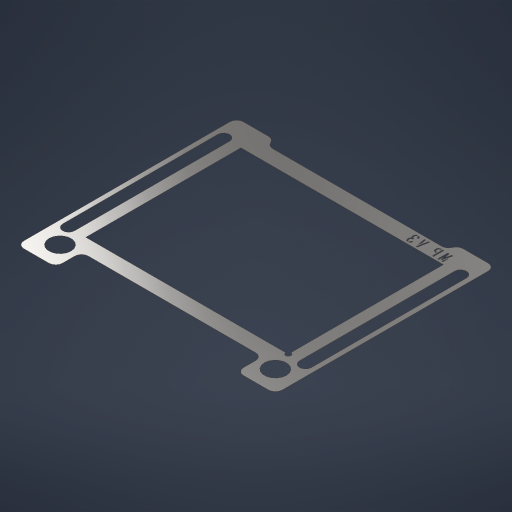
# Autodesk Inventor part: Module PCB Stencil - V3
Saved by Autodesk Inventor 2024 (Build 280153000, 153)
## iProperties
Created: 2022-06-23
Part Number: Module PCB Stencil - V3
Material: Stainless Steel
Document SubType Name: Modeling
Designer: Caleb
Density: 8 g/cm^3
Appearance: Semi-Polished
Author: Caleb
Autodesk Inventor part; units mm, degrees
ref_plane "YZ Plane" through (0, 0, 0) normal (1, 0, 0) x (0, 1, 0)
ref_plane "XZ Plane" through (0, 0, 0) normal (0, 1, 0) x (-1, 0, 0)
ref_plane "XY Plane" through (0, 0, 0) normal (0, 0, 1) x (1, 0, 0)
sketch "Sketch1" plane through (0, 0, 0) normal (0, 1, 0) x (-1, 0, 0)
  line L0 (-38.1, -34.925) -> (38.1, -34.925)
  line L1 (38.1, -34.925) -> (38.1, 34.925)
  line L2 (38.1, 34.925) -> (-38.1, 34.925)
  line L3 (-38.1, 34.925) -> (-38.1, -34.925)
  line L4 (-38.1, -34.925) -> (38.1, 34.925) construction
  line L5 (38.1, -34.925) -> (-38.1, 34.925) construction
  point P0 (0, 0)
  dimension "d0" = 76.2
  dimension "d1" = 69.85
  constraints: 12 end point, 2 midpoint, 2 parallel, 1 horizontal, 1 perpendicular
  measures "d0" distance of L2.end L1.end
  measures "d1" distance of L1.end L0.end
extrude "Extrusion1" add sketch "Sketch1" along normal blind 0.0508
sketch "Sketch2" plane through (0, 0.0508, 0) normal (0, 1, 0) x (1, 0, 0)
  line L0 (34.925, -22.86) -> (34.925, 22.86) construction
  line L1 (36.675, -22.86) -> (36.675, 22.86)
  line L2 (33.175, 22.86) -> (33.175, -22.86)
  arc A0 (33.175, -22.86) -> (36.675, -22.86) centre (34.925, -22.86) ccw
  arc A1 (36.675, 22.86) -> (33.175, 22.86) centre (34.925, 22.86) ccw
  line L3 (38.1, -34.925) -> (38.1, 34.925) projected
  line L4 (0, -11.2063) -> (0, 14.7333)
  line L5 (-34.925, -22.86) -> (-34.925, 22.86) construction
  line L6 (-36.675, -22.86) -> (-36.675, 22.86)
  line L7 (-33.175, 22.86) -> (-33.175, -22.86)
  arc A2 (-36.675, -22.86) -> (-33.175, -22.86) centre (-34.925, -22.86) ccw
  arc A3 (-33.175, 22.86) -> (-36.675, 22.86) centre (-34.925, 22.86) ccw
  line L8 (-38.1, -34.925) -> (38.1, -34.925) projected
  line L9 (-38.1, 34.925) -> (-38.1, -34.925) projected
  point P0 (0, 0)
  point P1 (34.925, 0)
  point P2 (-34.925, 0)
  point P3 (31.75, -28.575)
  point P4 (-31.75, -28.575)
  dimension "d4" = 3.5
  dimension "d5" = 3.175
  dimension "d6" = 45.72
  dimension "d14" = 6.35
  dimension "d15" = 6.35
  dimension "d16" = 6.35
  dimension "d17" = 6.35
  constraints: 18 end point, 8 point on circle, 7 symmetric about line, 4 centre point, 4 tangent, 2 vertical, 1 horizontal alignment, 1 midpoint, 1 parallel, 1 point on line, 2 other
  measures "d4" distance between parallel lines of L2 L1
  measures "d5" distance from line of L3 point (34.925, 0)
  measures "d6" distance of L0.end L0.start
  measures "d14" distance from line of L3 point (31.75, -28.575)
  measures "d15" distance from line of L8 point (31.75, -28.575)
  measures "d16" distance from line of L8 point (-31.75, -28.575)
  measures "d17" distance from line of L9 point (-31.75, -28.575)
extrude "Extrusion2" cut sketch "Sketch2" against normal through all
sketch "Sketch3" plane through (0, 0.0508, 0) normal (0, 1, 0) x (1, 0, 0)
  line L0 (-38.1, -34.925) -> (38.1, -34.925) projected
  line L1 (-26.67, -34.925) -> (26.67, -34.925)
  line L2 (26.67, -34.925) -> (26.67, -27.305)
  line L3 (26.67, -27.305) -> (-26.67, -27.305)
  line L4 (-26.67, -27.305) -> (-26.67, -34.925)
  line L5 (-38.1, 34.925) -> (-38.1, -34.925) projected
  line L6 (15.3292, 0) -> (-25.2672, 0)
  line L7 (-26.67, 34.925) -> (26.67, 34.925)
  line L8 (26.67, 34.925) -> (26.67, 27.305)
  line L9 (26.67, 27.305) -> (-26.67, 27.305)
  line L10 (-26.67, 27.305) -> (-26.67, 34.925)
  point P0 (0, 0)
  dimension "d9" = 7.62
  dimension "d10" = 53.34
  dimension "d11" = 11.43
  constraints: 18 end point, 4 symmetric about line, 2 horizontal, 2 parallel, 1 perpendicular, 1 point on line
  measures "d9" distance of L3.end L1.start
  measures "d10" distance between parallel lines of L4 L2
  measures "d11" distance between parallel lines of L5 L4
extrude "Extrusion3" cut sketch "Sketch3" against normal through all
sketch "Sketch4" plane through (0, 0.0508, 0) normal (0, 1, 0) x (1, 0, 0)
  line L0 (-38.1, 34.925) -> (-38.1, -34.925) projected
  line L1 (-38.1, -34.925) -> (-26.67, -34.925) projected
  line L2 (26.67, -34.925) -> (38.1, -34.925) projected
  line L3 (38.1, -34.925) -> (38.1, 34.925) projected
  point P0 (0, 0)
  point P1 (-31.75, -28.575)
  point P2 (31.75, -28.575)
  dimension "d18" = 6.35
  dimension "d19" = 6.35
  dimension "d20" = 6.35
  dimension "d21" = 6.35
  measures "d18" distance from line of L0 point (-31.75, -28.575)
  measures "d19" distance from line of L1 point (-31.75, -28.575)
  measures "d20" distance from line of L2 point (31.75, -28.575)
  measures "d21" distance from line of point (31.75, -28.575) L3
hole "Hole1" at (-31.75, 0.0508, 28.575) at (31.75, 0.0508, 28.575) direction (0, -1, 0) diameter 6.477 end through all
sketch "Sketch5" plane through (0, 0.0508, 0) normal (0, 1, 0) x (1, 0, 0)
  line L0 (-26.67, 34.925) -> (-38.1, 34.925) projected
  line L1 (38.1, -34.925) -> (38.1, 34.925) projected
  line L2 (-38.1, 34.925) -> (38.1, 34.925)
  line L3 (38.1, 34.925) -> (38.1, 29.845)
  line L4 (38.1, 29.845) -> (-38.1, 29.845)
  line L5 (-38.1, 29.845) -> (-38.1, 34.925)
  point P0 (0, 0)
  dimension "d29" = 5.08
  constraints: 8 end point, 2 parallel, 1 horizontal, 1 perpendicular, 1 point on line
  measures "d29" distance between parallel lines of L4 L2
extrude "Extrusion4" cut sketch "Sketch5" against normal through all
sketch "Sketch6" plane through (0, 0.0508, 0) normal (0, 1, 0) x (1, 0, 0)
  line L0 (-29.845, 22.86) -> (29.845, 22.86)
  line L1 (29.845, 22.86) -> (29.845, -22.86)
  line L2 (29.845, -22.86) -> (-29.845, -22.86)
  line L3 (-29.845, -22.86) -> (-29.845, 22.86)
  circle A0 centre (29.845, -22.86) radius 0.7938
  circle A1 centre (31.75, -28.575) radius 3.2385 projected
  point P0 (0, 0)
  point P1 (29.0512, -22.86)
  point P2 (29.845, -22.0662)
  dimension "d32" = 1.5875
  dimension "d33" = 45.72
  dimension "d34" = 59.69
  dimension "d38" = 5.715
  dimension "d39" = 1.905
  constraints: 8 end point, 2 parallel, 1 centre point, 1 coincident, 1 horizontal, 1 perpendicular
  measures "d32" diameter of A0
  measures "d33" distance of L2.end L0.start
  measures "d34" distance of L1.end L2.end
  measures "d38" distance from line of L2 A1.centre
  measures "d39" distance from line of L1 A1.centre
extrude "Extrusion5" cut sketch "Sketch6" against normal through all contours L0 L1 A0 L2 L3 | A0 L2 L1 | L1 L2 A0
fillet "Fillet1" radius 2 12 edges at (-26.67, 0.0254, 34.925) (-38.1, 0.0254, 34.925) (26.67, 0.0254, 34.925) (38.1, 0.0254, 34.925) (38.1, 0.0254, -29.845) (26.67, 0.0254, -29.845) (-26.67, 0.0254, -29.845) (-38.1, 0.0254, -29.845) (-26.67, 0.0254, -27.305) (26.67, 0.0254, -27.305) (-26.67, 0.0254, 27.305) (26.67, 0.0254, 27.305)
sketch "Sketch8" plane through (0, 0, 0) normal (0, -1, 0) x (1, 0, 0)
  line L0 (29.2698, -26.5478) -> (16.9198, -26.5478) construction
  line L1 (16.9198, -26.5478) -> (16.9198, -23.4808) construction
  line L2 (16.9198, -23.4808) -> (29.2698, -23.4808) construction
  line L3 (29.2698, -23.4808) -> (29.2698, -26.5478) construction
  line L4 (28.7006, -25.1078) -> (28.7006, -25.1205)
  line L5 (28.7006, -25.1205) -> (28.2949, -23.621)
  line L6 (28.2949, -23.621) -> (27.8956, -25.1333)
  line L7 (27.8956, -25.1333) -> (27.8914, -23.6253)
  spline S0 degree 2 poles (27.8914, -23.6253) (27.8914, -23.5615) (27.8107, -23.4851) (27.7384, -23.4808) knots 0 0 0 1 2 2 2
  line L8 (27.7384, -23.4808) -> (27.7002, -23.4808)
  spline S1 degree 2 poles (27.7002, -23.4808) (27.6237, -23.4829) (27.5388, -23.5658) (27.5388, -23.6295) knots 0 0 0 1 2 2 2
  line L9 (27.5388, -23.6295) -> (27.5388, -26.3821)
  spline S2 degree 2 poles (27.5388, -26.3821) (27.543, -26.4544) (27.6429, -26.5308) (27.7214, -26.5308) knots 0 0 0 1 2 2 2
  line L10 (27.7214, -26.5308) -> (27.7554, -26.5308)
  spline S3 degree 2 poles (27.7554, -26.5308) (27.8234, -26.5266) (27.9168, -26.4629) (27.9338, -26.4034) knots 0 0 0 1 2 2 2
  line L11 (27.9338, -26.4034) -> (28.3013, -24.9379)
  line L12 (28.3013, -24.9379) -> (28.6666, -26.4076)
  spline S4 degree 2 poles (28.6666, -26.4076) (28.6857, -26.4607) (28.7686, -26.5202) (28.8301, -26.5308) knots 0 0 0 1 2 2 2
  line L13 (28.8301, -26.5308) -> (28.9279, -26.5308)
  spline S5 degree 2 poles (28.9279, -26.5308) (28.9831, -26.5181) (29.0468, -26.4586) (29.0532, -26.4119) knots 0 0 0 1 2 2 2
  line L14 (29.0532, -26.4119) -> (28.7006, -25.1078)
  spline S6 degree 2 poles (29.0574, -23.6465) (29.0574, -23.5785) (28.9788, -23.4829) (28.9002, -23.4808) knots 0 0 0 1 2 2 2
  line L15 (28.9002, -23.4808) -> (28.8748, -23.4808)
  spline S7 degree 2 poles (28.8748, -23.4808) (28.8684, -23.4808) (28.862, -23.4808) knots 0 0 0 1 1 1
  spline S8 degree 2 poles (28.862, -23.4808) (28.7898, -23.4829) (28.7048, -23.5764) (28.7048, -23.6465) knots 0 0 0 1 2 2 2
  line L16 (28.7048, -23.6465) -> (28.7048, -23.8207)
  line L17 (28.7048, -23.8207) -> (29.0574, -25.1248)
  line L18 (29.0574, -25.1248) -> (29.0574, -23.6465)
  line L19 (26.1986, -23.4808) -> (26.1051, -23.4808)
  spline S9 degree 2 poles (26.1051, -23.4808) (26.052, -23.4829) (25.9777, -23.5467) (25.9756, -23.5934) knots 0 0 0 1 2 2 2
  line L20 (25.9756, -23.5934) -> (25.9756, -26.5436)
  line L21 (25.9756, -26.5436) -> (26.1986, -26.5436)
  spline S10 degree 2 poles (26.1986, -26.5436) (26.2517, -26.5414) (26.326, -26.4756) (26.3281, -26.4267) knots 0 0 0 1 2 2 2
  line L22 (26.3281, -26.4267) -> (26.3281, -23.5934)
  spline S11 degree 2 poles (26.3281, -23.5934) (26.326, -23.5467) (26.2517, -23.4829) (26.1986, -23.4808) knots 0 0 0 1 2 2 2
  line L23 (25.6272, -25.1418) -> (25.6272, -24.8423)
  line L24 (25.6272, -24.8423) -> (25.5401, -24.8423)
  spline S12 degree 2 poles (25.5401, -24.8423) (25.3554, -24.8423) (25.0049, -24.9952) (24.7691, -25.2777) (24.7543, -25.4773) knots 0 0 0 1 2 3 3 3
  spline S13 degree 2 poles (24.7543, -25.4773) (24.7479, -25.6855) (24.7543, -25.8958) knots 0 0 0 1 1 1
  spline S14 degree 2 poles (24.7543, -25.8958) (24.7649, -26.0954) (25.0007, -26.3843) (25.3554, -26.5414) (25.5401, -26.5436) knots 0 0 0 1 2 3 3 3
  line L25 (25.5401, -26.5436) -> (25.6272, -26.5436)
  line L26 (25.6272, -26.5436) -> (25.6272, -26.2398)
  line L27 (25.6272, -26.2398) -> (25.5316, -26.2398)
  spline S15 degree 2 poles (25.5316, -26.2398) (25.3511, -26.2356) (25.1154, -26.0274) (25.1111, -25.8703) knots 0 0 0 1 2 2 2
  spline S16 degree 2 poles (25.1111, -25.8703) (25.1026, -25.7811) (25.109, -25.6027) (25.1111, -25.5113) knots 0 0 0 1 2 2 2
  spline S17 degree 2 poles (25.1111, -25.5113) (25.1154, -25.3584) (25.3511, -25.146) (25.5316, -25.1418) knots 0 0 0 1 2 2 2
  line L28 (25.5316, -25.1418) -> (25.6272, -25.1418)
  line L29 (22.1078, -26.4777) -> (21.5429, -23.5509)
  spline S18 degree 2 poles (21.5429, -23.5509) (21.528, -23.4999) (21.4813, -23.4787) (21.4473, -23.4808) knots 0 0 0 1 2 2 2
  line L30 (21.4473, -23.4808) -> (21.254, -23.4808)
  spline S19 degree 2 poles (21.254, -23.4808) (21.2328, -23.4808) (21.203, -23.4851) (21.1903, -23.4936) knots 0 0 0 1 2 2 2
  line L31 (21.1903, -23.4936) -> (21.5386, -25.3393)
  line L32 (21.5386, -25.3393) -> (21.7595, -26.4862)
  spline S20 degree 2 poles (21.7595, -26.4862) (21.7659, -26.5202) (21.7935, -26.5414) (21.8253, -26.5436) knots 0 0 0 1 2 2 2
  line L33 (21.8253, -26.5436) -> (22.042, -26.5436)
  spline S21 degree 2 poles (22.042, -26.5436) (22.0781, -26.5436) (22.1142, -26.516) (22.1078, -26.4777) knots 0 0 0 1 2 2 2
  line L34 (21.0076, -24.3771) -> (20.6019, -26.4692)
  spline S22 degree 2 poles (20.6019, -26.4692) (20.5956, -26.5117) (20.6211, -26.5436) (20.6508, -26.5436) knots 0 0 0 1 2 2 2
  line L35 (20.6508, -26.5436) -> (20.8674, -26.5436)
  spline S23 degree 2 poles (20.8674, -26.5436) (20.8972, -26.5436) (20.9397, -26.516) (20.9503, -26.4735) knots 0 0 0 1 2 2 2
  line L36 (20.9503, -26.4735) -> (21.1775, -25.2947)
  line L37 (21.1775, -25.2947) -> (21.0076, -24.3771)
  spline S24 degree 2 poles (18.7456, -24.855) (18.6394, -24.855) (18.4504, -24.7637) (18.3293, -24.598) (18.3272, -24.4897) knots 0 0 0 1 2 3 3 3
  line L38 (18.3272, -24.4897) -> (18.3272, -24.1308)
  spline S25 degree 2 poles (18.3272, -24.1308) (18.3293, -24.0203) (18.461, -23.844) (18.5714, -23.7994) knots 0 0 0 1 2 2 2
  line L39 (18.5714, -23.7994) -> (18.5714, -23.4808)
  spline S26 degree 2 poles (18.5714, -23.4808) (18.3973, -23.5169) (18.1318, -23.7102) (17.981, -23.9842) (17.9789, -24.1392) knots 0 0 0 1 2 3 3 3
  line L40 (17.9789, -24.1392) -> (17.9789, -24.4791)
  spline S27 degree 2 poles (17.9789, -24.4791) (17.981, -24.6384) (18.136, -24.9166) (18.2741, -25.0164) knots 0 0 0 1 2 2 2
  spline S28 degree 2 poles (18.2741, -25.0164) (18.136, -25.1141) (17.981, -25.3924) (17.9789, -25.5474) knots 0 0 0 1 2 2 2
  line L41 (17.9789, -25.5474) -> (17.9789, -25.8915)
  spline S29 degree 2 poles (17.9789, -25.8915) (17.981, -26.0466) (18.136, -26.3163) (18.4015, -26.5096) (18.5714, -26.5478) knots 0 0 0 1 2 3 3 3
  line L42 (18.5714, -26.5478) -> (18.5714, -26.2313)
  spline S30 degree 2 poles (18.5714, -26.2313) (18.461, -26.1825) (18.3293, -26.0083) (18.3272, -25.8958) knots 0 0 0 1 2 2 2
  line L43 (18.3272, -25.8958) -> (18.3272, -25.5389)
  spline S31 degree 2 poles (18.3272, -25.5389) (18.3293, -25.4285) (18.4525, -25.2649) (18.6415, -25.1736) (18.7456, -25.1736) knots 0 0 0 1 2 3 3 3
  spline S32 degree 2 poles (18.7456, -25.1736) (18.8518, -25.1736) (18.9219, -25.1375) (18.9176, -25.095) knots 0 0 0 1 2 2 2
  line L44 (18.9176, -25.095) -> (18.9176, -25.0164)
  spline S33 degree 2 poles (18.9176, -25.0164) (18.9198, -24.9655) (18.9176, -24.8933) (18.8454, -24.855) (18.7456, -24.855) knots 0 0 0 1 2 3 3 3
  line L45 (19.5102, -25.9425) -> (19.5102, -25.8915)
  spline S34 degree 2 poles (19.5102, -25.8915) (19.5124, -25.8193) (19.472, -25.7789) (19.4062, -25.7832) knots 0 0 0 1 2 2 2
  spline S35 degree 2 poles (19.4062, -25.7832) (19.3892, -25.7832) (19.3552, -25.7832) (19.3361, -25.7832) knots 0 0 0 1 2 2 2
  spline S36 degree 2 poles (19.3361, -25.7832) (19.3042, -25.7832) (19.283, -25.7832) knots 0 0 0 1 1 1
  spline S37 degree 2 poles (19.283, -25.7832) (19.2023, -25.7789) (19.1577, -25.8193) (19.1577, -25.8958) knots 0 0 0 1 2 2 2
  spline S38 degree 2 poles (19.1577, -25.8958) (19.1555, -26.0083) (19.0281, -26.1825) (18.9176, -26.2313) knots 0 0 0 1 2 2 2
  line L46 (18.9176, -26.2313) -> (18.9176, -26.5478)
  spline S39 degree 2 poles (18.9176, -26.5478) (19.164, -26.4905) (19.4869, -26.1634) (19.5102, -25.9425) knots 0 0 0 1 2 2 2
  spline S40 degree 2 poles (18.9134, -23.4808) (18.9176, -23.4872) (18.9176, -23.4999) (18.9176, -23.5063) knots 0 0 0 1 2 2 2
  line L47 (18.9176, -23.5063) -> (18.9176, -23.8037)
  spline S41 degree 2 poles (18.9176, -23.8037) (19.0281, -23.8461) (19.1555, -24.0203) (19.1577, -24.1329) knots 0 0 0 1 2 2 2
  spline S42 degree 2 poles (19.1577, -24.1329) (19.1555, -24.2051) (19.1874, -24.2497) (19.2405, -24.2454) knots 0 0 0 1 2 2 2
  spline S43 degree 2 poles (19.2405, -24.2454) (19.2723, -24.2454) (19.3318, -24.2454) knots 0 0 0 1 1 1
  spline S44 degree 2 poles (19.3318, -24.2454) (19.3573, -24.2454) (19.3998, -24.2454) (19.4189, -24.2454) knots 0 0 0 1 2 2 2
  spline S45 degree 2 poles (19.4189, -24.2454) (19.4762, -24.2497) (19.5124, -24.2115) (19.5102, -24.1414) knots 0 0 0 1 2 2 2
  spline S46 degree 2 poles (19.5102, -24.1414) (19.5081, -23.9863) (19.3573, -23.7145) (19.0897, -23.5191) (18.9134, -23.4808) knots 0 0 0 1 2 3 3 3
  point P0 (0, 0)
  dimension "d0" = 76.2
  dimension "d1" = 69.85
  constraints: 2 other
emboss "Emboss2" sketch "Sketch8" operation cut depth 1 direction (0, 1, 0)
equation "\"d15\" = d14"
equation "\"d16\" = d14"
equation "\"d17\" = d14"
equation "\"d19\" = d18"
equation "\"d20\" = d18"
equation "\"d21\" = d18"
body "Solid1"
